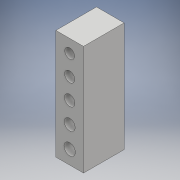
# Autodesk Inventor part: Screw size Test
Saved by Autodesk Inventor 2017 (Build 210142000, 142)
## iProperties
Created: 2017-05-18
Part Number: Screw size Test
Material: Generic
Document SubType Name: Modeling
Designer: Lillian
Density: 1 g/cm^3
Appearance: Default
Author: Lillian
Autodesk Inventor part; units mm, degrees
ref_plane "YZ Plane" through (0, 0, 0) normal (1, 0, 0) x (0, 1, 0)
ref_plane "XZ Plane" through (0, 0, 0) normal (0, 1, 0) x (-1, 0, 0)
ref_plane "XY Plane" through (0, 0, 0) normal (0, 0, 1) x (1, 0, 0)
sketch "Sketch1" plane through (0, 0, 0) normal (0, 1, 0) x (-1, 0, 0)
  circle A0 centre (0, 0) radius 1.3
  circle A1 centre (0, 5.05) radius 1.25
  circle A2 centre (0, -5.15) radius 1.35
  line L0 (3.4, 13.2) -> (-3.4, 13.2)
  line L1 (-3.4, 13.2) -> (-3.4, -13.8)
  line L2 (-3.4, -13.8) -> (3.4, -13.8)
  line L3 (3.4, -13.8) -> (3.4, 13.2)
  circle A3 centre (0, -10.4) radius 1.4
  circle A4 centre (0, 10) radius 1.2
  dimension "d0" = 2.6
  dimension "d1" = 2.5
  dimension "d2" = 2.5
  dimension "d3" = 2.5
  dimension "d4" = 2.7
  dimension "d5" = 2.5
  dimension "d6" = 2.5
  dimension "d7" = 2.8
  dimension "d8" = 2.4
  dimension "d9" = 2
  dimension "d10" = 2
  dimension "d11" = 2
  dimension "d12" = 2
  constraints: 8 end point, 5 centre point, 2 parallel, 1 coincident, 1 horizontal, 1 perpendicular
  measures "d0" diameter of A0
  measures "d3" diameter of A1
  measures "d4" diameter of A2
  measures "d7" diameter of A3
  measures "d8" diameter of A4
  measures "d9" distance edge to line of A3 L3
  measures "d10" distance edge to line of A3 L1
  measures "d11" distance edge to line of A3 L2
  measures "d12" distance edge to line of A4 L0
extrude "Extrusion1" add sketch "Sketch1" along normal blind 10
sketch "Sketch2" plane through (0, 10, 0) normal (0, 1, 0) x (1, 0, 0)
  line L0 (-2.0805, -11.7201) -> (2.1464, -11.7201) construction
  line L1 (2.1464, -11.7201) -> (2.1464, -12.7412) construction
  line L2 (2.1464, -12.7412) -> (-2.0805, -12.7412) construction
  line L3 (-2.0805, -12.7412) -> (-2.0805, -11.7201) construction
  line L4 (-1.0805, -10.7201) -> (3.1464, -10.7201) construction
  line L5 (3.1464, -10.7201) -> (3.1464, -11.7412) construction
  line L6 (3.1464, -11.7412) -> (-1.0805, -11.7412) construction
  line L7 (-1.0805, -11.7412) -> (-1.0805, -10.7201) construction
  line L8 (-1.8538, -6.831) -> (2.3732, -6.831) construction
  line L9 (2.3732, -6.831) -> (2.3732, -7.852) construction
  line L10 (2.3732, -7.852) -> (-1.8538, -7.852) construction
  line L11 (-1.8538, -7.852) -> (-1.8538, -6.831) construction
  line L12 (-1.9, -1.8736) -> (2.3269, -1.8736) construction
  line L13 (2.3269, -1.8736) -> (2.3269, -2.8947) construction
  line L14 (2.3269, -2.8947) -> (-1.9, -2.8947) construction
  line L15 (-1.9, -2.8947) -> (-1.9, -1.8736) construction
  line L16 (-1.934, 2.8467) -> (2.2929, 2.8467) construction
  line L17 (2.2929, 2.8467) -> (2.2929, 1.8257) construction
  line L18 (2.2929, 1.8257) -> (-1.934, 1.8257) construction
  line L19 (-1.934, 1.8257) -> (-1.934, 2.8467) construction
  line L20 (-1.7841, 8.3554) -> (2.4428, 8.3554) construction
  line L21 (2.4428, 8.3554) -> (2.4428, 7.3343) construction
  line L22 (2.4428, 7.3343) -> (-1.7841, 7.3343) construction
  line L23 (-1.7841, 7.3343) -> (-1.7841, 8.3554) construction
  line L24 (-1.3908, -12.7412) -> (-2.0075, -12.7412)
  line L25 (-2.0075, -12.7412) -> (-2.0075, -12.5994)
  spline S0 degree 2 poles (-2.0075, -12.5994) (-1.9411, -12.537) (-1.8228, -12.4211) (-1.766, -12.3587) knots 0 0 0 1 2 2 2
  spline S1 degree 2 poles (-1.766, -12.3587) (-1.6518, -12.2331) (-1.5683, -12.0824) (-1.5683, -12.0021) knots 0 0 0 1 2 2 2
  spline S2 degree 2 poles (-1.5683, -12.0021) (-1.5683, -11.96) (-1.5942, -11.8968) (-1.6177, -11.8765) knots 0 0 0 1 2 2 2
  spline S3 degree 2 poles (-1.6177, -11.8765) (-1.6413, -11.8563) (-1.7028, -11.836) (-1.7401, -11.836) knots 0 0 0 1 2 2 2
  spline S4 degree 2 poles (-1.7401, -11.836) (-1.7758, -11.836) (-1.8487, -11.8538) (-1.8819, -11.8676) knots 0 0 0 1 2 2 2
  spline S5 degree 2 poles (-1.8819, -11.8676) (-1.9103, -11.879) (-1.963, -11.9114) (-1.9792, -11.9227) knots 0 0 0 1 2 2 2
  line L26 (-1.9792, -11.9227) -> (-1.9865, -11.9227)
  line L27 (-1.9865, -11.9227) -> (-1.9865, -11.7801)
  spline S6 degree 2 poles (-1.9865, -11.7801) (-1.9451, -11.7598) (-1.7968, -11.7201) (-1.7304, -11.7201) knots 0 0 0 1 2 2 2
  spline S7 degree 2 poles (-1.7304, -11.7201) (-1.5902, -11.7201) (-1.4322, -11.8684) (-1.4322, -11.9948) knots 0 0 0 1 2 2 2
  spline S8 degree 2 poles (-1.4322, -11.9948) (-1.4322, -12.054) (-1.4597, -12.1529) (-1.484, -12.195) knots 0 0 0 1 2 2 2
  spline S9 degree 2 poles (-1.484, -12.195) (-1.5083, -12.2388) (-1.5789, -12.3247) (-1.6177, -12.366) knots 0 0 0 1 2 2 2
  spline S10 degree 2 poles (-1.6177, -12.366) (-1.681, -12.4349) (-1.8357, -12.5824) (-1.8819, -12.6253) knots 0 0 0 1 2 2 2
  line L28 (-1.8819, -12.6253) -> (-1.3908, -12.6253)
  line L29 (-1.3908, -12.6253) -> (-1.3908, -12.7412)
  line L30 (-1.0424, -12.7412) -> (-1.2028, -12.7412)
  line L31 (-1.2028, -12.7412) -> (-1.2028, -12.5499)
  line L32 (-1.2028, -12.5499) -> (-1.0424, -12.5499)
  line L33 (-1.0424, -12.5499) -> (-1.0424, -12.7412)
  line L34 (-0.1972, -12.3976) -> (-0.3163, -12.3976)
  line L35 (-0.3163, -12.3976) -> (-0.3163, -12.7412)
  line L36 (-0.3163, -12.7412) -> (-0.4451, -12.7412)
  line L37 (-0.4451, -12.7412) -> (-0.4451, -12.3976)
  line L38 (-0.4451, -12.3976) -> (-0.8868, -12.3976)
  line L39 (-0.8868, -12.3976) -> (-0.8868, -12.2566)
  line L40 (-0.8868, -12.2566) -> (-0.4395, -11.7412)
  line L41 (-0.4395, -11.7412) -> (-0.3163, -11.7412)
  line L42 (-0.3163, -11.7412) -> (-0.3163, -12.2898)
  line L43 (-0.3163, -12.2898) -> (-0.1972, -12.2898)
  line L44 (-0.1972, -12.2898) -> (-0.1972, -12.3976)
  line L45 (-0.4451, -12.2898) -> (-0.4451, -11.8992)
  line L46 (-0.4451, -11.8992) -> (-0.7814, -12.2898)
  line L47 (-0.7814, -12.2898) -> (-0.4451, -12.2898)
  line L48 (0.7793, -12.7412) -> (0.7793, -12.3068)
  spline S11 degree 2 poles (0.7793, -12.3068) (0.7793, -12.255) (0.7712, -12.1666) (0.7583, -12.1423) knots 0 0 0 1 2 2 2
  spline S12 degree 2 poles (0.7583, -12.1423) (0.7453, -12.1156) (0.6959, -12.0897) (0.6529, -12.0897) knots 0 0 0 1 2 2 2
  spline S13 degree 2 poles (0.6529, -12.0897) (0.614, -12.0897) (0.5249, -12.1375) (0.4779, -12.1828) knots 0 0 0 1 2 2 2
  spline S14 degree 2 poles (0.4779, -12.1828) (0.4787, -12.1942) (0.4803, -12.2258) (0.4803, -12.2469) knots 0 0 0 1 2 2 2
  line L49 (0.4803, -12.2469) -> (0.4803, -12.7412)
  line L50 (0.4803, -12.7412) -> (0.3539, -12.7412)
  line L51 (0.3539, -12.7412) -> (0.3539, -12.3068)
  spline S15 degree 2 poles (0.3539, -12.3068) (0.3539, -12.255) (0.3458, -12.1666) (0.3328, -12.1423) knots 0 0 0 1 2 2 2
  spline S16 degree 2 poles (0.3328, -12.1423) (0.3199, -12.1156) (0.2704, -12.0897) (0.2275, -12.0897) knots 0 0 0 1 2 2 2
  spline S17 degree 2 poles (0.2275, -12.0897) (0.187, -12.0897) (0.097, -12.1407) (0.0549, -12.1804) knots 0 0 0 1 2 2 2
  line L52 (0.0549, -12.1804) -> (0.0549, -12.7412)
  line L53 (0.0549, -12.7412) -> (-0.0716, -12.7412)
  line L54 (-0.0716, -12.7412) -> (-0.0716, -11.9908)
  line L55 (-0.0716, -11.9908) -> (0.0549, -11.9908)
  line L56 (0.0549, -11.9908) -> (0.0549, -12.0734)
  spline S18 degree 2 poles (0.0549, -12.0734) (0.1043, -12.024) (0.2015, -11.9697) (0.2599, -11.9697) knots 0 0 0 1 2 2 2
  spline S19 degree 2 poles (0.2599, -11.9697) (0.3263, -11.9697) (0.4293, -12.0305) (0.456, -12.0994) knots 0 0 0 1 2 2 2
  spline S20 degree 2 poles (0.456, -12.0994) (0.5135, -12.0354) (0.6221, -11.9697) (0.6853, -11.9697) knots 0 0 0 1 2 2 2
  spline S21 degree 2 poles (0.6853, -11.9697) (0.734, -11.9697) (0.8134, -11.9997) (0.8425, -12.0337) knots 0 0 0 1 2 2 2
  spline S22 degree 2 poles (0.8425, -12.0337) (0.8725, -12.0678) (0.9058, -12.1699) (0.9058, -12.2469) knots 0 0 0 1 2 2 2
  line L57 (0.9058, -12.2469) -> (0.9058, -12.7412)
  line L58 (0.9058, -12.7412) -> (0.7793, -12.7412)
  line L59 (1.9341, -12.7412) -> (1.9341, -12.3068)
  spline S23 degree 2 poles (1.9341, -12.3068) (1.9341, -12.255) (1.926, -12.1666) (1.913, -12.1423) knots 0 0 0 1 2 2 2
  spline S24 degree 2 poles (1.913, -12.1423) (1.9001, -12.1156) (1.8506, -12.0897) (1.8077, -12.0897) knots 0 0 0 1 2 2 2
  spline S25 degree 2 poles (1.8077, -12.0897) (1.7688, -12.0897) (1.6797, -12.1375) (1.6327, -12.1828) knots 0 0 0 1 2 2 2
  spline S26 degree 2 poles (1.6327, -12.1828) (1.6335, -12.1942) (1.6351, -12.2258) (1.6351, -12.2469) knots 0 0 0 1 2 2 2
  line L60 (1.6351, -12.2469) -> (1.6351, -12.7412)
  line L61 (1.6351, -12.7412) -> (1.5087, -12.7412)
  line L62 (1.5087, -12.7412) -> (1.5087, -12.3068)
  spline S27 degree 2 poles (1.5087, -12.3068) (1.5087, -12.255) (1.5006, -12.1666) (1.4876, -12.1423) knots 0 0 0 1 2 2 2
  spline S28 degree 2 poles (1.4876, -12.1423) (1.4746, -12.1156) (1.4252, -12.0897) (1.3823, -12.0897) knots 0 0 0 1 2 2 2
  spline S29 degree 2 poles (1.3823, -12.0897) (1.3417, -12.0897) (1.2518, -12.1407) (1.2096, -12.1804) knots 0 0 0 1 2 2 2
  line L63 (1.2096, -12.1804) -> (1.2096, -12.7412)
  line L64 (1.2096, -12.7412) -> (1.0832, -12.7412)
  line L65 (1.0832, -12.7412) -> (1.0832, -11.9908)
  line L66 (1.0832, -11.9908) -> (1.2096, -11.9908)
  line L67 (1.2096, -11.9908) -> (1.2096, -12.0734)
  spline S30 degree 2 poles (1.2096, -12.0734) (1.2591, -12.024) (1.3563, -11.9697) (1.4147, -11.9697) knots 0 0 0 1 2 2 2
  spline S31 degree 2 poles (1.4147, -11.9697) (1.4811, -11.9697) (1.584, -12.0305) (1.6108, -12.0994) knots 0 0 0 1 2 2 2
  spline S32 degree 2 poles (1.6108, -12.0994) (1.6683, -12.0354) (1.7769, -11.9697) (1.8401, -11.9697) knots 0 0 0 1 2 2 2
  spline S33 degree 2 poles (1.8401, -11.9697) (1.8887, -11.9697) (1.9682, -11.9997) (1.9973, -12.0337) knots 0 0 0 1 2 2 2
  spline S34 degree 2 poles (1.9973, -12.0337) (2.0273, -12.0678) (2.0605, -12.1699) (2.0605, -12.2469) knots 0 0 0 1 2 2 2
  line L68 (2.0605, -12.2469) -> (2.0605, -12.7412)
  line L69 (2.0605, -12.7412) -> (1.9341, -12.7412)
  line L70 (-1.1641, -7.852) -> (-1.7808, -7.852)
  line L71 (-1.7808, -7.852) -> (-1.7808, -7.7102)
  spline S35 degree 2 poles (-1.7808, -7.7102) (-1.7144, -7.6478) (-1.5961, -7.5319) (-1.5393, -7.4695) knots 0 0 0 1 2 2 2
  spline S36 degree 2 poles (-1.5393, -7.4695) (-1.4251, -7.3439) (-1.3416, -7.1932) (-1.3416, -7.113) knots 0 0 0 1 2 2 2
  spline S37 degree 2 poles (-1.3416, -7.113) (-1.3416, -7.0708) (-1.3675, -7.0076) (-1.391, -6.9874) knots 0 0 0 1 2 2 2
  spline S38 degree 2 poles (-1.391, -6.9874) (-1.4145, -6.9671) (-1.4761, -6.9469) (-1.5134, -6.9469) knots 0 0 0 1 2 2 2
  spline S39 degree 2 poles (-1.5134, -6.9469) (-1.5491, -6.9469) (-1.622, -6.9647) (-1.6552, -6.9785) knots 0 0 0 1 2 2 2
  spline S40 degree 2 poles (-1.6552, -6.9785) (-1.6836, -6.9898) (-1.7363, -7.0222) (-1.7525, -7.0336) knots 0 0 0 1 2 2 2
  line L72 (-1.7525, -7.0336) -> (-1.7598, -7.0336)
  line L73 (-1.7598, -7.0336) -> (-1.7598, -6.8909)
  spline S41 degree 2 poles (-1.7598, -6.8909) (-1.7184, -6.8707) (-1.5701, -6.831) (-1.5037, -6.831) knots 0 0 0 1 2 2 2
  spline S42 degree 2 poles (-1.5037, -6.831) (-1.3635, -6.831) (-1.2055, -6.9793) (-1.2055, -7.1057) knots 0 0 0 1 2 2 2
  spline S43 degree 2 poles (-1.2055, -7.1057) (-1.2055, -7.1648) (-1.233, -7.2637) (-1.2573, -7.3058) knots 0 0 0 1 2 2 2
  spline S44 degree 2 poles (-1.2573, -7.3058) (-1.2816, -7.3496) (-1.3521, -7.4355) (-1.391, -7.4768) knots 0 0 0 1 2 2 2
  spline S45 degree 2 poles (-1.391, -7.4768) (-1.4542, -7.5457) (-1.609, -7.6932) (-1.6552, -7.7362) knots 0 0 0 1 2 2 2
  line L74 (-1.6552, -7.7362) -> (-1.1641, -7.7362)
  line L75 (-1.1641, -7.7362) -> (-1.1641, -7.852)
  line L76 (-0.8157, -7.852) -> (-0.9761, -7.852)
  line L77 (-0.9761, -7.852) -> (-0.9761, -7.6608)
  line L78 (-0.9761, -7.6608) -> (-0.8157, -7.6608)
  line L79 (-0.8157, -7.6608) -> (-0.8157, -7.852)
  spline S46 degree 2 poles (-0.0077, -7.5344) (-0.0077, -7.6065) (-0.0539, -7.7297) (-0.0961, -7.7751) knots 0 0 0 1 2 2 2
  spline S47 degree 2 poles (-0.0961, -7.7751) (-0.1382, -7.8204) (-0.2638, -7.8731) (-0.3416, -7.8731) knots 0 0 0 1 2 2 2
  spline S48 degree 2 poles (-0.3416, -7.8731) (-0.4129, -7.8731) (-0.5523, -7.8415) (-0.6033, -7.8164) knots 0 0 0 1 2 2 2
  line L80 (-0.6033, -7.8164) -> (-0.6033, -7.6746)
  line L81 (-0.6033, -7.6746) -> (-0.5936, -7.6746)
  spline S49 degree 2 poles (-0.5936, -7.6746) (-0.5782, -7.6859) (-0.5207, -7.7151) (-0.4858, -7.7281) knots 0 0 0 1 2 2 2
  spline S50 degree 2 poles (-0.4858, -7.7281) (-0.4461, -7.7418) (-0.3805, -7.7572) (-0.3392, -7.7572) knots 0 0 0 1 2 2 2
  spline S51 degree 2 poles (-0.3392, -7.7572) (-0.2986, -7.7572) (-0.2225, -7.7281) (-0.1949, -7.6964) knots 0 0 0 1 2 2 2
  spline S52 degree 2 poles (-0.1949, -7.6964) (-0.1698, -7.6665) (-0.1439, -7.587) (-0.1439, -7.5336) knots 0 0 0 1 2 2 2
  spline S53 degree 2 poles (-0.1439, -7.5336) (-0.1439, -7.4801) (-0.173, -7.412) (-0.2006, -7.3893) knots 0 0 0 1 2 2 2
  spline S54 degree 2 poles (-0.2006, -7.3893) (-0.229, -7.3642) (-0.3132, -7.3431) (-0.3643, -7.3431) knots 0 0 0 1 2 2 2
  spline S55 degree 2 poles (-0.3643, -7.3431) (-0.4194, -7.3431) (-0.5288, -7.3601) (-0.562, -7.3674) knots 0 0 0 1 2 2 2
  line L82 (-0.562, -7.3674) -> (-0.562, -6.852)
  line L83 (-0.562, -6.852) -> (-0.0134, -6.852)
  line L84 (-0.0134, -6.852) -> (-0.0134, -6.9695)
  line L85 (-0.0134, -6.9695) -> (-0.4332, -6.9695)
  line L86 (-0.4332, -6.9695) -> (-0.4332, -7.2362)
  spline S56 degree 2 poles (-0.4332, -7.2362) (-0.4089, -7.2329) (-0.3619, -7.2305) (-0.3424, -7.2305) knots 0 0 0 1 2 2 2
  spline S57 degree 2 poles (-0.3424, -7.2305) (-0.2654, -7.2305) (-0.1593, -7.2556) (-0.1106, -7.2929) knots 0 0 0 1 2 2 2
  spline S58 degree 2 poles (-0.1106, -7.2929) (-0.0612, -7.3302) (-0.0077, -7.4436) (-0.0077, -7.5344) knots 0 0 0 1 2 2 2
  line L87 (1.0061, -7.852) -> (1.0061, -7.4177)
  spline S59 degree 2 poles (1.0061, -7.4177) (1.0061, -7.3658) (0.9979, -7.2775) (0.985, -7.2532) knots 0 0 0 1 2 2 2
  spline S60 degree 2 poles (0.985, -7.2532) (0.972, -7.2264) (0.9226, -7.2005) (0.8796, -7.2005) knots 0 0 0 1 2 2 2
  spline S61 degree 2 poles (0.8796, -7.2005) (0.8407, -7.2005) (0.7516, -7.2483) (0.7046, -7.2937) knots 0 0 0 1 2 2 2
  spline S62 degree 2 poles (0.7046, -7.2937) (0.7054, -7.305) (0.707, -7.3366) (0.707, -7.3577) knots 0 0 0 1 2 2 2
  line L88 (0.707, -7.3577) -> (0.707, -7.852)
  line L89 (0.707, -7.852) -> (0.5806, -7.852)
  line L90 (0.5806, -7.852) -> (0.5806, -7.4177)
  spline S63 degree 2 poles (0.5806, -7.4177) (0.5806, -7.3658) (0.5725, -7.2775) (0.5595, -7.2532) knots 0 0 0 1 2 2 2
  spline S64 degree 2 poles (0.5595, -7.2532) (0.5466, -7.2264) (0.4971, -7.2005) (0.4542, -7.2005) knots 0 0 0 1 2 2 2
  spline S65 degree 2 poles (0.4542, -7.2005) (0.4137, -7.2005) (0.3237, -7.2516) (0.2816, -7.2913) knots 0 0 0 1 2 2 2
  line L91 (0.2816, -7.2913) -> (0.2816, -7.852)
  line L92 (0.2816, -7.852) -> (0.1552, -7.852)
  line L93 (0.1552, -7.852) -> (0.1552, -7.1016)
  line L94 (0.1552, -7.1016) -> (0.2816, -7.1016)
  line L95 (0.2816, -7.1016) -> (0.2816, -7.1843)
  spline S66 degree 2 poles (0.2816, -7.1843) (0.331, -7.1349) (0.4283, -7.0806) (0.4866, -7.0806) knots 0 0 0 1 2 2 2
  spline S67 degree 2 poles (0.4866, -7.0806) (0.5531, -7.0806) (0.656, -7.1413) (0.6827, -7.2102) knots 0 0 0 1 2 2 2
  spline S68 degree 2 poles (0.6827, -7.2102) (0.7402, -7.1462) (0.8488, -7.0806) (0.912, -7.0806) knots 0 0 0 1 2 2 2
  spline S69 degree 2 poles (0.912, -7.0806) (0.9607, -7.0806) (1.0401, -7.1105) (1.0693, -7.1446) knots 0 0 0 1 2 2 2
  spline S70 degree 2 poles (1.0693, -7.1446) (1.0992, -7.1786) (1.1325, -7.2807) (1.1325, -7.3577) knots 0 0 0 1 2 2 2
  line L96 (1.1325, -7.3577) -> (1.1325, -7.852)
  line L97 (1.1325, -7.852) -> (1.0061, -7.852)
  line L98 (2.1608, -7.852) -> (2.1608, -7.4177)
  spline S71 degree 2 poles (2.1608, -7.4177) (2.1608, -7.3658) (2.1527, -7.2775) (2.1398, -7.2532) knots 0 0 0 1 2 2 2
  spline S72 degree 2 poles (2.1398, -7.2532) (2.1268, -7.2264) (2.0774, -7.2005) (2.0344, -7.2005) knots 0 0 0 1 2 2 2
  spline S73 degree 2 poles (2.0344, -7.2005) (1.9955, -7.2005) (1.9064, -7.2483) (1.8594, -7.2937) knots 0 0 0 1 2 2 2
  spline S74 degree 2 poles (1.8594, -7.2937) (1.8602, -7.305) (1.8618, -7.3366) (1.8618, -7.3577) knots 0 0 0 1 2 2 2
  line L99 (1.8618, -7.3577) -> (1.8618, -7.852)
  line L100 (1.8618, -7.852) -> (1.7354, -7.852)
  line L101 (1.7354, -7.852) -> (1.7354, -7.4177)
  spline S75 degree 2 poles (1.7354, -7.4177) (1.7354, -7.3658) (1.7273, -7.2775) (1.7143, -7.2532) knots 0 0 0 1 2 2 2
  spline S76 degree 2 poles (1.7143, -7.2532) (1.7014, -7.2264) (1.6519, -7.2005) (1.609, -7.2005) knots 0 0 0 1 2 2 2
  spline S77 degree 2 poles (1.609, -7.2005) (1.5685, -7.2005) (1.4785, -7.2516) (1.4364, -7.2913) knots 0 0 0 1 2 2 2
  line L102 (1.4364, -7.2913) -> (1.4364, -7.852)
  line L103 (1.4364, -7.852) -> (1.3099, -7.852)
  line L104 (1.3099, -7.852) -> (1.3099, -7.1016)
  line L105 (1.3099, -7.1016) -> (1.4364, -7.1016)
  line L106 (1.4364, -7.1016) -> (1.4364, -7.1843)
  spline S78 degree 2 poles (1.4364, -7.1843) (1.4858, -7.1349) (1.583, -7.0806) (1.6414, -7.0806) knots 0 0 0 1 2 2 2
  spline S79 degree 2 poles (1.6414, -7.0806) (1.7078, -7.0806) (1.8108, -7.1413) (1.8375, -7.2102) knots 0 0 0 1 2 2 2
  spline S80 degree 2 poles (1.8375, -7.2102) (1.895, -7.1462) (2.0036, -7.0806) (2.0668, -7.0806) knots 0 0 0 1 2 2 2
  spline S81 degree 2 poles (2.0668, -7.0806) (2.1155, -7.0806) (2.1949, -7.1105) (2.224, -7.1446) knots 0 0 0 1 2 2 2
  spline S82 degree 2 poles (2.224, -7.1446) (2.254, -7.1786) (2.2873, -7.2807) (2.2873, -7.3577) knots 0 0 0 1 2 2 2
  line L107 (2.2873, -7.3577) -> (2.2873, -7.852)
  line L108 (2.2873, -7.852) -> (2.1608, -7.852)
  line L109 (-1.2103, -2.8947) -> (-1.827, -2.8947)
  line L110 (-1.827, -2.8947) -> (-1.827, -2.7528)
  spline S83 degree 2 poles (-1.827, -2.7528) (-1.7606, -2.6904) (-1.6423, -2.5746) (-1.5855, -2.5122) knots 0 0 0 1 2 2 2
  spline S84 degree 2 poles (-1.5855, -2.5122) (-1.4713, -2.3866) (-1.3878, -2.2358) (-1.3878, -2.1556) knots 0 0 0 1 2 2 2
  spline S85 degree 2 poles (-1.3878, -2.1556) (-1.3878, -2.1135) (-1.4137, -2.0502) (-1.4372, -2.03) knots 0 0 0 1 2 2 2
  spline S86 degree 2 poles (-1.4372, -2.03) (-1.4607, -2.0097) (-1.5223, -1.9895) (-1.5596, -1.9895) knots 0 0 0 1 2 2 2
  spline S87 degree 2 poles (-1.5596, -1.9895) (-1.5953, -1.9895) (-1.6682, -2.0073) (-1.7014, -2.0211) knots 0 0 0 1 2 2 2
  spline S88 degree 2 poles (-1.7014, -2.0211) (-1.7298, -2.0324) (-1.7825, -2.0648) (-1.7987, -2.0762) knots 0 0 0 1 2 2 2
  line L111 (-1.7987, -2.0762) -> (-1.806, -2.0762)
  line L112 (-1.806, -2.0762) -> (-1.806, -1.9336)
  spline S89 degree 2 poles (-1.806, -1.9336) (-1.7646, -1.9133) (-1.6163, -1.8736) (-1.5499, -1.8736) knots 0 0 0 1 2 2 2
  spline S90 degree 2 poles (-1.5499, -1.8736) (-1.4097, -1.8736) (-1.2517, -2.0219) (-1.2517, -2.1483) knots 0 0 0 1 2 2 2
  spline S91 degree 2 poles (-1.2517, -2.1483) (-1.2517, -2.2075) (-1.2792, -2.3063) (-1.3035, -2.3485) knots 0 0 0 1 2 2 2
  spline S92 degree 2 poles (-1.3035, -2.3485) (-1.3278, -2.3922) (-1.3983, -2.4781) (-1.4372, -2.5195) knots 0 0 0 1 2 2 2
  spline S93 degree 2 poles (-1.4372, -2.5195) (-1.5004, -2.5883) (-1.6552, -2.7358) (-1.7014, -2.7788) knots 0 0 0 1 2 2 2
  line L113 (-1.7014, -2.7788) -> (-1.2103, -2.7788)
  line L114 (-1.2103, -2.7788) -> (-1.2103, -2.8947)
  line L115 (-0.8619, -2.8947) -> (-1.0223, -2.8947)
  line L116 (-1.0223, -2.8947) -> (-1.0223, -2.7034)
  line L117 (-1.0223, -2.7034) -> (-0.8619, -2.7034)
  line L118 (-0.8619, -2.7034) -> (-0.8619, -2.8947)
  spline S94 degree 2 poles (-0.028, -2.5705) (-0.028, -2.6475) (-0.0791, -2.778) (-0.122, -2.8217) knots 0 0 0 1 2 2 2
  spline S95 degree 2 poles (-0.122, -2.8217) (-0.1666, -2.8679) (-0.2784, -2.9157) (-0.3457, -2.9157) knots 0 0 0 1 2 2 2
  spline S96 degree 2 poles (-0.3457, -2.9157) (-0.4129, -2.9157) (-0.5239, -2.8703) (-0.5661, -2.825) knots 0 0 0 1 2 2 2
  spline S97 degree 2 poles (-0.5661, -2.825) (-0.6179, -2.7707) (-0.6763, -2.5883) (-0.6763, -2.4554) knots 0 0 0 1 2 2 2
  spline S98 degree 2 poles (-0.6763, -2.4554) (-0.6763, -2.325) (-0.6228, -2.1151) (-0.5669, -2.0373) knots 0 0 0 1 2 2 2
  spline S99 degree 2 poles (-0.5669, -2.0373) (-0.5126, -1.9611) (-0.3408, -1.876) (-0.2282, -1.876) knots 0 0 0 1 2 2 2
  spline S100 degree 2 poles (-0.2282, -1.876) (-0.1949, -1.876) (-0.1366, -1.8825) (-0.1147, -1.8898) knots 0 0 0 1 2 2 2
  line L119 (-0.1147, -1.8898) -> (-0.1147, -2.0186)
  line L120 (-0.1147, -2.0186) -> (-0.1204, -2.0186)
  spline S101 degree 2 poles (-0.1204, -2.0186) (-0.139, -2.0089) (-0.2071, -1.9919) (-0.246, -1.9919) knots 0 0 0 1 2 2 2
  spline S102 degree 2 poles (-0.246, -1.9919) (-0.3708, -1.9919) (-0.5239, -2.1605) (-0.5385, -2.3258) knots 0 0 0 1 2 2 2
  spline S103 degree 2 poles (-0.5385, -2.3258) (-0.4907, -2.2925) (-0.3902, -2.2561) (-0.3303, -2.2561) knots 0 0 0 1 2 2 2
  spline S104 degree 2 poles (-0.3303, -2.2561) (-0.2719, -2.2561) (-0.1844, -2.2796) (-0.1366, -2.3152) knots 0 0 0 1 2 2 2
  spline S105 degree 2 poles (-0.1366, -2.3152) (-0.0815, -2.3566) (-0.028, -2.4846) (-0.028, -2.5705) knots 0 0 0 1 2 2 2
  spline S106 degree 2 poles (-0.1641, -2.5762) (-0.1641, -2.5146) (-0.1966, -2.4311) (-0.2322, -2.4019) knots 0 0 0 1 2 2 2
  spline S107 degree 2 poles (-0.2322, -2.4019) (-0.259, -2.3809) (-0.3254, -2.3671) (-0.3603, -2.3671) knots 0 0 0 1 2 2 2
  spline S108 degree 2 poles (-0.3603, -2.3671) (-0.4073, -2.3671) (-0.4956, -2.3955) (-0.5385, -2.4222) knots 0 0 0 1 2 2 2
  spline S109 degree 2 poles (-0.5385, -2.4222) (-0.5393, -2.4368) (-0.541, -2.4643) (-0.541, -2.4854) knots 0 0 0 1 2 2 2
  spline S110 degree 2 poles (-0.541, -2.4854) (-0.541, -2.5891) (-0.5004, -2.7164) (-0.4697, -2.7496) knots 0 0 0 1 2 2 2
  spline S111 degree 2 poles (-0.4697, -2.7496) (-0.4413, -2.7812) (-0.3797, -2.8063) (-0.3449, -2.8063) knots 0 0 0 1 2 2 2
  spline S112 degree 2 poles (-0.3449, -2.8063) (-0.2638, -2.8063) (-0.1641, -2.6913) (-0.1641, -2.5762) knots 0 0 0 1 2 2 2
  line L121 (0.9598, -2.8947) -> (0.9598, -2.4603)
  spline S113 degree 2 poles (0.9598, -2.4603) (0.9598, -2.4084) (0.9517, -2.3201) (0.9388, -2.2958) knots 0 0 0 1 2 2 2
  spline S114 degree 2 poles (0.9388, -2.2958) (0.9258, -2.269) (0.8764, -2.2431) (0.8334, -2.2431) knots 0 0 0 1 2 2 2
  spline S115 degree 2 poles (0.8334, -2.2431) (0.7945, -2.2431) (0.7054, -2.2909) (0.6584, -2.3363) knots 0 0 0 1 2 2 2
  spline S116 degree 2 poles (0.6584, -2.3363) (0.6592, -2.3477) (0.6608, -2.3793) (0.6608, -2.4003) knots 0 0 0 1 2 2 2
  line L122 (0.6608, -2.4003) -> (0.6608, -2.8947)
  line L123 (0.6608, -2.8947) -> (0.5344, -2.8947)
  line L124 (0.5344, -2.8947) -> (0.5344, -2.4603)
  spline S117 degree 2 poles (0.5344, -2.4603) (0.5344, -2.4084) (0.5263, -2.3201) (0.5133, -2.2958) knots 0 0 0 1 2 2 2
  spline S118 degree 2 poles (0.5133, -2.2958) (0.5004, -2.269) (0.4509, -2.2431) (0.408, -2.2431) knots 0 0 0 1 2 2 2
  spline S119 degree 2 poles (0.408, -2.2431) (0.3675, -2.2431) (0.2775, -2.2942) (0.2354, -2.3339) knots 0 0 0 1 2 2 2
  line L125 (0.2354, -2.3339) -> (0.2354, -2.8947)
  line L126 (0.2354, -2.8947) -> (0.109, -2.8947)
  line L127 (0.109, -2.8947) -> (0.109, -2.1443)
  line L128 (0.109, -2.1443) -> (0.2354, -2.1443)
  line L129 (0.2354, -2.1443) -> (0.2354, -2.2269)
  spline S120 degree 2 poles (0.2354, -2.2269) (0.2848, -2.1775) (0.3821, -2.1232) (0.4404, -2.1232) knots 0 0 0 1 2 2 2
  spline S121 degree 2 poles (0.4404, -2.1232) (0.5068, -2.1232) (0.6098, -2.184) (0.6365, -2.2528) knots 0 0 0 1 2 2 2
  spline S122 degree 2 poles (0.6365, -2.2528) (0.694, -2.1888) (0.8026, -2.1232) (0.8658, -2.1232) knots 0 0 0 1 2 2 2
  spline S123 degree 2 poles (0.8658, -2.1232) (0.9145, -2.1232) (0.9939, -2.1532) (1.0231, -2.1872) knots 0 0 0 1 2 2 2
  spline S124 degree 2 poles (1.0231, -2.1872) (1.053, -2.2212) (1.0863, -2.3233) (1.0863, -2.4003) knots 0 0 0 1 2 2 2
  line L130 (1.0863, -2.4003) -> (1.0863, -2.8947)
  line L131 (1.0863, -2.8947) -> (0.9598, -2.8947)
  line L132 (2.1146, -2.8947) -> (2.1146, -2.4603)
  spline S125 degree 2 poles (2.1146, -2.4603) (2.1146, -2.4084) (2.1065, -2.3201) (2.0936, -2.2958) knots 0 0 0 1 2 2 2
  spline S126 degree 2 poles (2.0936, -2.2958) (2.0806, -2.269) (2.0312, -2.2431) (1.9882, -2.2431) knots 0 0 0 1 2 2 2
  spline S127 degree 2 poles (1.9882, -2.2431) (1.9493, -2.2431) (1.8602, -2.2909) (1.8132, -2.3363) knots 0 0 0 1 2 2 2
  spline S128 degree 2 poles (1.8132, -2.3363) (1.814, -2.3477) (1.8156, -2.3793) (1.8156, -2.4003) knots 0 0 0 1 2 2 2
  line L133 (1.8156, -2.4003) -> (1.8156, -2.8947)
  line L134 (1.8156, -2.8947) -> (1.6892, -2.8947)
  line L135 (1.6892, -2.8947) -> (1.6892, -2.4603)
  spline S129 degree 2 poles (1.6892, -2.4603) (1.6892, -2.4084) (1.6811, -2.3201) (1.6681, -2.2958) knots 0 0 0 1 2 2 2
  spline S130 degree 2 poles (1.6681, -2.2958) (1.6551, -2.269) (1.6057, -2.2431) (1.5628, -2.2431) knots 0 0 0 1 2 2 2
  spline S131 degree 2 poles (1.5628, -2.2431) (1.5222, -2.2431) (1.4323, -2.2942) (1.3902, -2.3339) knots 0 0 0 1 2 2 2
  line L136 (1.3902, -2.3339) -> (1.3902, -2.8947)
  line L137 (1.3902, -2.8947) -> (1.2637, -2.8947)
  line L138 (1.2637, -2.8947) -> (1.2637, -2.1443)
  line L139 (1.2637, -2.1443) -> (1.3902, -2.1443)
  line L140 (1.3902, -2.1443) -> (1.3902, -2.2269)
  spline S132 degree 2 poles (1.3902, -2.2269) (1.4396, -2.1775) (1.5368, -2.1232) (1.5952, -2.1232) knots 0 0 0 1 2 2 2
  spline S133 degree 2 poles (1.5952, -2.1232) (1.6616, -2.1232) (1.7645, -2.184) (1.7913, -2.2528) knots 0 0 0 1 2 2 2
  spline S134 degree 2 poles (1.7913, -2.2528) (1.8488, -2.1888) (1.9574, -2.1232) (2.0206, -2.1232) knots 0 0 0 1 2 2 2
  spline S135 degree 2 poles (2.0206, -2.1232) (2.0692, -2.1232) (2.1487, -2.1532) (2.1778, -2.1872) knots 0 0 0 1 2 2 2
  spline S136 degree 2 poles (2.1778, -2.1872) (2.2078, -2.2212) (2.241, -2.3233) (2.241, -2.4003) knots 0 0 0 1 2 2 2
  line L141 (2.241, -2.4003) -> (2.241, -2.8947)
  line L142 (2.241, -2.8947) -> (2.1146, -2.8947)
  line L143 (-1.2444, 1.8257) -> (-1.8611, 1.8257)
  line L144 (-1.8611, 1.8257) -> (-1.8611, 1.9675)
  spline S137 degree 2 poles (-1.8611, 1.9675) (-1.7946, 2.0299) (-1.6763, 2.1458) (-1.6196, 2.2082) knots 0 0 0 1 2 2 2
  spline S138 degree 2 poles (-1.6196, 2.2082) (-1.5053, 2.3338) (-1.4218, 2.4845) (-1.4218, 2.5647) knots 0 0 0 1 2 2 2
  spline S139 degree 2 poles (-1.4218, 2.5647) (-1.4218, 2.6069) (-1.4478, 2.6701) (-1.4713, 2.6903) knots 0 0 0 1 2 2 2
  spline S140 degree 2 poles (-1.4713, 2.6903) (-1.4948, 2.7106) (-1.5564, 2.7309) (-1.5936, 2.7309) knots 0 0 0 1 2 2 2
  spline S141 degree 2 poles (-1.5936, 2.7309) (-1.6293, 2.7309) (-1.7022, 2.713) (-1.7354, 2.6993) knots 0 0 0 1 2 2 2
  spline S142 degree 2 poles (-1.7354, 2.6993) (-1.7638, 2.6879) (-1.8165, 2.6555) (-1.8327, 2.6442) knots 0 0 0 1 2 2 2
  line L145 (-1.8327, 2.6442) -> (-1.84, 2.6442)
  line L146 (-1.84, 2.6442) -> (-1.84, 2.7868)
  spline S143 degree 2 poles (-1.84, 2.7868) (-1.7987, 2.807) (-1.6504, 2.8467) (-1.5839, 2.8467) knots 0 0 0 1 2 2 2
  spline S144 degree 2 poles (-1.5839, 2.8467) (-1.4437, 2.8467) (-1.2857, 2.6984) (-1.2857, 2.572) knots 0 0 0 1 2 2 2
  spline S145 degree 2 poles (-1.2857, 2.572) (-1.2857, 2.5129) (-1.3132, 2.414) (-1.3376, 2.3719) knots 0 0 0 1 2 2 2
  spline S146 degree 2 poles (-1.3376, 2.3719) (-1.3619, 2.3281) (-1.4324, 2.2422) (-1.4713, 2.2009) knots 0 0 0 1 2 2 2
  spline S147 degree 2 poles (-1.4713, 2.2009) (-1.5345, 2.132) (-1.6893, 1.9845) (-1.7354, 1.9416) knots 0 0 0 1 2 2 2
  line L147 (-1.7354, 1.9416) -> (-1.2444, 1.9416)
  line L148 (-1.2444, 1.9416) -> (-1.2444, 1.8257)
  line L149 (-0.8959, 1.8257) -> (-1.0564, 1.8257)
  line L150 (-1.0564, 1.8257) -> (-1.0564, 2.0169)
  line L151 (-1.0564, 2.0169) -> (-0.8959, 2.0169)
  line L152 (-0.8959, 2.0169) -> (-0.8959, 1.8257)
  line L153 (-0.0661, 2.6758) -> (-0.4988, 1.8257)
  line L154 (-0.4988, 1.8257) -> (-0.6414, 1.8257)
  line L155 (-0.6414, 1.8257) -> (-0.1844, 2.7082)
  line L156 (-0.1844, 2.7082) -> (-0.7006, 2.7082)
  line L157 (-0.7006, 2.7082) -> (-0.7006, 2.8257)
  line L158 (-0.7006, 2.8257) -> (-0.0661, 2.8257)
  line L159 (-0.0661, 2.8257) -> (-0.0661, 2.6758)
  line L160 (0.9258, 1.8257) -> (0.9258, 2.26)
  spline S148 degree 2 poles (0.9258, 2.26) (0.9258, 2.3119) (0.9177, 2.4002) (0.9047, 2.4245) knots 0 0 0 1 2 2 2
  spline S149 degree 2 poles (0.9047, 2.4245) (0.8918, 2.4513) (0.8423, 2.4772) (0.7994, 2.4772) knots 0 0 0 1 2 2 2
  spline S150 degree 2 poles (0.7994, 2.4772) (0.7605, 2.4772) (0.6714, 2.4294) (0.6244, 2.384) knots 0 0 0 1 2 2 2
  spline S151 degree 2 poles (0.6244, 2.384) (0.6252, 2.3727) (0.6268, 2.3411) (0.6268, 2.32) knots 0 0 0 1 2 2 2
  line L161 (0.6268, 2.32) -> (0.6268, 1.8257)
  line L162 (0.6268, 1.8257) -> (0.5004, 1.8257)
  line L163 (0.5004, 1.8257) -> (0.5004, 2.26)
  spline S152 degree 2 poles (0.5004, 2.26) (0.5004, 2.3119) (0.4923, 2.4002) (0.4793, 2.4245) knots 0 0 0 1 2 2 2
  spline S153 degree 2 poles (0.4793, 2.4245) (0.4663, 2.4513) (0.4169, 2.4772) (0.374, 2.4772) knots 0 0 0 1 2 2 2
  spline S154 degree 2 poles (0.374, 2.4772) (0.3334, 2.4772) (0.2435, 2.4262) (0.2013, 2.3865) knots 0 0 0 1 2 2 2
  line L164 (0.2013, 2.3865) -> (0.2013, 1.8257)
  line L165 (0.2013, 1.8257) -> (0.0749, 1.8257)
  line L166 (0.0749, 1.8257) -> (0.0749, 2.5761)
  line L167 (0.0749, 2.5761) -> (0.2013, 2.5761)
  line L168 (0.2013, 2.5761) -> (0.2013, 2.4934)
  spline S155 degree 2 poles (0.2013, 2.4934) (0.2508, 2.5429) (0.348, 2.5972) (0.4064, 2.5972) knots 0 0 0 1 2 2 2
  spline S156 degree 2 poles (0.4064, 2.5972) (0.4728, 2.5972) (0.5757, 2.5364) (0.6025, 2.4675) knots 0 0 0 1 2 2 2
  spline S157 degree 2 poles (0.6025, 2.4675) (0.66, 2.5315) (0.7686, 2.5972) (0.8318, 2.5972) knots 0 0 0 1 2 2 2
  spline S158 degree 2 poles (0.8318, 2.5972) (0.8804, 2.5972) (0.9599, 2.5672) (0.989, 2.5331) knots 0 0 0 1 2 2 2
  spline S159 degree 2 poles (0.989, 2.5331) (1.019, 2.4991) (1.0522, 2.397) (1.0522, 2.32) knots 0 0 0 1 2 2 2
  line L169 (1.0522, 2.32) -> (1.0522, 1.8257)
  line L170 (1.0522, 1.8257) -> (0.9258, 1.8257)
  line L171 (2.0806, 1.8257) -> (2.0806, 2.26)
  spline S160 degree 2 poles (2.0806, 2.26) (2.0806, 2.3119) (2.0725, 2.4002) (2.0595, 2.4245) knots 0 0 0 1 2 2 2
  spline S161 degree 2 poles (2.0595, 2.4245) (2.0466, 2.4513) (1.9971, 2.4772) (1.9542, 2.4772) knots 0 0 0 1 2 2 2
  spline S162 degree 2 poles (1.9542, 2.4772) (1.9153, 2.4772) (1.8261, 2.4294) (1.7791, 2.384) knots 0 0 0 1 2 2 2
  spline S163 degree 2 poles (1.7791, 2.384) (1.7799, 2.3727) (1.7816, 2.3411) (1.7816, 2.32) knots 0 0 0 1 2 2 2
  line L172 (1.7816, 2.32) -> (1.7816, 1.8257)
  line L173 (1.7816, 1.8257) -> (1.6552, 1.8257)
  line L174 (1.6552, 1.8257) -> (1.6552, 2.26)
  spline S164 degree 2 poles (1.6552, 2.26) (1.6552, 2.3119) (1.647, 2.4002) (1.6341, 2.4245) knots 0 0 0 1 2 2 2
  spline S165 degree 2 poles (1.6341, 2.4245) (1.6211, 2.4513) (1.5717, 2.4772) (1.5287, 2.4772) knots 0 0 0 1 2 2 2
  spline S166 degree 2 poles (1.5287, 2.4772) (1.4882, 2.4772) (1.3983, 2.4262) (1.3561, 2.3865) knots 0 0 0 1 2 2 2
  line L175 (1.3561, 2.3865) -> (1.3561, 1.8257)
  line L176 (1.3561, 1.8257) -> (1.2297, 1.8257)
  line L177 (1.2297, 1.8257) -> (1.2297, 2.5761)
  line L178 (1.2297, 2.5761) -> (1.3561, 2.5761)
  line L179 (1.3561, 2.5761) -> (1.3561, 2.4934)
  spline S167 degree 2 poles (1.3561, 2.4934) (1.4056, 2.5429) (1.5028, 2.5972) (1.5611, 2.5972) knots 0 0 0 1 2 2 2
  spline S168 degree 2 poles (1.5611, 2.5972) (1.6276, 2.5972) (1.7305, 2.5364) (1.7573, 2.4675) knots 0 0 0 1 2 2 2
  spline S169 degree 2 poles (1.7573, 2.4675) (1.8148, 2.5315) (1.9234, 2.5972) (1.9866, 2.5972) knots 0 0 0 1 2 2 2
  spline S170 degree 2 poles (1.9866, 2.5972) (2.0352, 2.5972) (2.1146, 2.5672) (2.1438, 2.5331) knots 0 0 0 1 2 2 2
  spline S171 degree 2 poles (2.1438, 2.5331) (2.1738, 2.4991) (2.207, 2.397) (2.207, 2.32) knots 0 0 0 1 2 2 2
  line L180 (2.207, 2.32) -> (2.207, 1.8257)
  line L181 (2.207, 1.8257) -> (2.0806, 1.8257)
  line L182 (-1.0945, 7.3327) -> (-1.7112, 7.3327)
  line L183 (-1.7112, 7.3327) -> (-1.7112, 7.4745)
  spline S172 degree 2 poles (-1.7112, 7.4745) (-1.6448, 7.5369) (-1.5264, 7.6528) (-1.4697, 7.7152) knots 0 0 0 1 2 2 2
  spline S173 degree 2 poles (-1.4697, 7.7152) (-1.3554, 7.8408) (-1.272, 7.9915) (-1.272, 8.0717) knots 0 0 0 1 2 2 2
  spline S174 degree 2 poles (-1.272, 8.0717) (-1.272, 8.1139) (-1.2979, 8.1771) (-1.3214, 8.1973) knots 0 0 0 1 2 2 2
  spline S175 degree 2 poles (-1.3214, 8.1973) (-1.3449, 8.2176) (-1.4065, 8.2378) (-1.4438, 8.2378) knots 0 0 0 1 2 2 2
  spline S176 degree 2 poles (-1.4438, 8.2378) (-1.4794, 8.2378) (-1.5524, 8.22) (-1.5856, 8.2062) knots 0 0 0 1 2 2 2
  spline S177 degree 2 poles (-1.5856, 8.2062) (-1.614, 8.1949) (-1.6666, 8.1625) (-1.6828, 8.1511) knots 0 0 0 1 2 2 2
  line L184 (-1.6828, 8.1511) -> (-1.6901, 8.1511)
  line L185 (-1.6901, 8.1511) -> (-1.6901, 8.2938)
  spline S178 degree 2 poles (-1.6901, 8.2938) (-1.6488, 8.314) (-1.5005, 8.3537) (-1.4341, 8.3537) knots 0 0 0 1 2 2 2
  spline S179 degree 2 poles (-1.4341, 8.3537) (-1.2939, 8.3537) (-1.1358, 8.2054) (-1.1358, 8.079) knots 0 0 0 1 2 2 2
  spline S180 degree 2 poles (-1.1358, 8.079) (-1.1358, 8.0199) (-1.1634, 7.921) (-1.1877, 7.8789) knots 0 0 0 1 2 2 2
  spline S181 degree 2 poles (-1.1877, 7.8789) (-1.212, 7.8351) (-1.2825, 7.7492) (-1.3214, 7.7079) knots 0 0 0 1 2 2 2
  spline S182 degree 2 poles (-1.3214, 7.7079) (-1.3846, 7.639) (-1.5394, 7.4915) (-1.5856, 7.4485) knots 0 0 0 1 2 2 2
  line L186 (-1.5856, 7.4485) -> (-1.0945, 7.4485)
  line L187 (-1.0945, 7.4485) -> (-1.0945, 7.3327)
  line L188 (-0.746, 7.3327) -> (-0.9065, 7.3327)
  line L189 (-0.9065, 7.3327) -> (-0.9065, 7.5239)
  line L190 (-0.9065, 7.5239) -> (-0.746, 7.5239)
  line L191 (-0.746, 7.5239) -> (-0.746, 7.3327)
  spline S183 degree 2 poles (-0.242, 7.31) (-0.3166, 7.31) (-0.4389, 7.3545) (-0.4819, 7.3959) knots 0 0 0 1 2 2 2
  spline S184 degree 2 poles (-0.4819, 7.3959) (-0.524, 7.4364) (-0.5678, 7.5466) (-0.5678, 7.609) knots 0 0 0 1 2 2 2
  spline S185 degree 2 poles (-0.5678, 7.609) (-0.5678, 7.69) (-0.4811, 7.8262) (-0.3984, 7.8667) knots 0 0 0 1 2 2 2
  line L192 (-0.3984, 7.8667) -> (-0.3984, 7.8708)
  spline S186 degree 2 poles (-0.3984, 7.8708) (-0.4721, 7.9137) (-0.5435, 8.0158) (-0.5435, 8.092) knots 0 0 0 1 2 2 2
  spline S187 degree 2 poles (-0.5435, 8.092) (-0.5435, 8.2046) (-0.3733, 8.3554) (-0.242, 8.3554) knots 0 0 0 1 2 2 2
  spline S188 degree 2 poles (-0.242, 8.3554) (-0.1059, 8.3554) (0.0587, 8.2127) (0.0587, 8.1009) knots 0 0 0 1 2 2 2
  spline S189 degree 2 poles (0.0587, 8.1009) (0.0587, 8.0336) (-0.02, 7.9024) (-0.0937, 7.8651) knots 0 0 0 1 2 2 2
  line L193 (-0.0937, 7.8651) -> (-0.0937, 7.861)
  spline S190 degree 2 poles (-0.0937, 7.861) (-0.0062, 7.8205) (0.0838, 7.7038) (0.0838, 7.6114) knots 0 0 0 1 2 2 2
  spline S191 degree 2 poles (0.0838, 7.6114) (0.0838, 7.4834) (-0.1026, 7.31) (-0.242, 7.31) knots 0 0 0 1 2 2 2
  spline S192 degree 2 poles (-0.054, 7.5985) (-0.054, 7.6601) (-0.1026, 7.733) (-0.1715, 7.7703) knots 0 0 0 1 2 2 2
  spline S193 degree 2 poles (-0.1715, 7.7703) (-0.1942, 7.7832) (-0.2704, 7.8132) (-0.3182, 7.8327) knots 0 0 0 1 2 2 2
  spline S194 degree 2 poles (-0.3182, 7.8327) (-0.3733, 7.7962) (-0.4324, 7.6876) (-0.4324, 7.6187) knots 0 0 0 1 2 2 2
  spline S195 degree 2 poles (-0.4324, 7.6187) (-0.4324, 7.528) (-0.323, 7.4096) (-0.2404, 7.4096) knots 0 0 0 1 2 2 2
  spline S196 degree 2 poles (-0.2404, 7.4096) (-0.1561, 7.4096) (-0.054, 7.5109) (-0.054, 7.5985) knots 0 0 0 1 2 2 2
  spline S197 degree 2 poles (-0.0726, 8.0993) (-0.0726, 8.1665) (-0.1626, 8.2565) (-0.2428, 8.2565) knots 0 0 0 1 2 2 2
  spline S198 degree 2 poles (-0.2428, 8.2565) (-0.3157, 8.2565) (-0.4089, 8.1763) (-0.4089, 8.1074) knots 0 0 0 1 2 2 2
  spline S199 degree 2 poles (-0.4089, 8.1074) (-0.4089, 8.0579) (-0.3611, 7.9891) (-0.3133, 7.9615) knots 0 0 0 1 2 2 2
  spline S200 degree 2 poles (-0.3133, 7.9615) (-0.293, 7.9502) (-0.2072, 7.9105) (-0.1723, 7.8991) knots 0 0 0 1 2 2 2
  spline S201 degree 2 poles (-0.1723, 7.8991) (-0.114, 7.9437) (-0.0726, 8.0385) (-0.0726, 8.0993) knots 0 0 0 1 2 2 2
  line L194 (1.0757, 7.3327) -> (1.0757, 7.767)
  spline S202 degree 2 poles (1.0757, 7.767) (1.0757, 7.8189) (1.0676, 7.9072) (1.0546, 7.9315) knots 0 0 0 1 2 2 2
  spline S203 degree 2 poles (1.0546, 7.9315) (1.0416, 7.9583) (0.9922, 7.9842) (0.9493, 7.9842) knots 0 0 0 1 2 2 2
  spline S204 degree 2 poles (0.9493, 7.9842) (0.9104, 7.9842) (0.8212, 7.9364) (0.7742, 7.891) knots 0 0 0 1 2 2 2
  spline S205 degree 2 poles (0.7742, 7.891) (0.775, 7.8797) (0.7766, 7.8481) (0.7766, 7.827) knots 0 0 0 1 2 2 2
  line L195 (0.7766, 7.827) -> (0.7766, 7.3327)
  line L196 (0.7766, 7.3327) -> (0.6502, 7.3327)
  line L197 (0.6502, 7.3327) -> (0.6502, 7.767)
  spline S206 degree 2 poles (0.6502, 7.767) (0.6502, 7.8189) (0.6421, 7.9072) (0.6292, 7.9315) knots 0 0 0 1 2 2 2
  spline S207 degree 2 poles (0.6292, 7.9315) (0.6162, 7.9583) (0.5668, 7.9842) (0.5238, 7.9842) knots 0 0 0 1 2 2 2
  spline S208 degree 2 poles (0.5238, 7.9842) (0.4833, 7.9842) (0.3933, 7.9331) (0.3512, 7.8934) knots 0 0 0 1 2 2 2
  line L198 (0.3512, 7.8934) -> (0.3512, 7.3327)
  line L199 (0.3512, 7.3327) -> (0.2248, 7.3327)
  line L200 (0.2248, 7.3327) -> (0.2248, 8.0831)
  line L201 (0.2248, 8.0831) -> (0.3512, 8.0831)
  line L202 (0.3512, 8.0831) -> (0.3512, 8.0004)
  spline S209 degree 2 poles (0.3512, 8.0004) (0.4006, 8.0498) (0.4979, 8.1041) (0.5562, 8.1041) knots 0 0 0 1 2 2 2
  spline S210 degree 2 poles (0.5562, 8.1041) (0.6227, 8.1041) (0.7256, 8.0434) (0.7523, 7.9745) knots 0 0 0 1 2 2 2
  spline S211 degree 2 poles (0.7523, 7.9745) (0.8099, 8.0385) (0.9185, 8.1041) (0.9817, 8.1041) knots 0 0 0 1 2 2 2
  spline S212 degree 2 poles (0.9817, 8.1041) (1.0303, 8.1041) (1.1097, 8.0742) (1.1389, 8.0401) knots 0 0 0 1 2 2 2
  spline S213 degree 2 poles (1.1389, 8.0401) (1.1689, 8.0061) (1.2021, 7.904) (1.2021, 7.827) knots 0 0 0 1 2 2 2
  line L203 (1.2021, 7.827) -> (1.2021, 7.3327)
  line L204 (1.2021, 7.3327) -> (1.0757, 7.3327)
  line L205 (2.2305, 7.3327) -> (2.2305, 7.767)
  spline S214 degree 2 poles (2.2305, 7.767) (2.2305, 7.8189) (2.2223, 7.9072) (2.2094, 7.9315) knots 0 0 0 1 2 2 2
  spline S215 degree 2 poles (2.2094, 7.9315) (2.1964, 7.9583) (2.147, 7.9842) (2.104, 7.9842) knots 0 0 0 1 2 2 2
  spline S216 degree 2 poles (2.104, 7.9842) (2.0651, 7.9842) (1.976, 7.9364) (1.929, 7.891) knots 0 0 0 1 2 2 2
  spline S217 degree 2 poles (1.929, 7.891) (1.9298, 7.8797) (1.9314, 7.8481) (1.9314, 7.827) knots 0 0 0 1 2 2 2
  line L206 (1.9314, 7.827) -> (1.9314, 7.3327)
  line L207 (1.9314, 7.3327) -> (1.805, 7.3327)
  line L208 (1.805, 7.3327) -> (1.805, 7.767)
  spline S218 degree 2 poles (1.805, 7.767) (1.805, 7.8189) (1.7969, 7.9072) (1.7839, 7.9315) knots 0 0 0 1 2 2 2
  spline S219 degree 2 poles (1.7839, 7.9315) (1.771, 7.9583) (1.7215, 7.9842) (1.6786, 7.9842) knots 0 0 0 1 2 2 2
  spline S220 degree 2 poles (1.6786, 7.9842) (1.6381, 7.9842) (1.5481, 7.9331) (1.506, 7.8934) knots 0 0 0 1 2 2 2
  line L209 (1.506, 7.8934) -> (1.506, 7.3327)
  line L210 (1.506, 7.3327) -> (1.3796, 7.3327)
  line L211 (1.3796, 7.3327) -> (1.3796, 8.0831)
  line L212 (1.3796, 8.0831) -> (1.506, 8.0831)
  line L213 (1.506, 8.0831) -> (1.506, 8.0004)
  spline S221 degree 2 poles (1.506, 8.0004) (1.5554, 8.0498) (1.6527, 8.1041) (1.711, 8.1041) knots 0 0 0 1 2 2 2
  spline S222 degree 2 poles (1.711, 8.1041) (1.7775, 8.1041) (1.8804, 8.0434) (1.9071, 7.9745) knots 0 0 0 1 2 2 2
  spline S223 degree 2 poles (1.9071, 7.9745) (1.9646, 8.0385) (2.0732, 8.1041) (2.1364, 8.1041) knots 0 0 0 1 2 2 2
  spline S224 degree 2 poles (2.1364, 8.1041) (2.1851, 8.1041) (2.2645, 8.0742) (2.2937, 8.0401) knots 0 0 0 1 2 2 2
  spline S225 degree 2 poles (2.2937, 8.0401) (2.3236, 8.0061) (2.3569, 7.904) (2.3569, 7.827) knots 0 0 0 1 2 2 2
  line L214 (2.3569, 7.827) -> (2.3569, 7.3327)
  line L215 (2.3569, 7.3327) -> (2.2305, 7.3327)
  point P0 (0, 0)
  constraints: 11 other
extrude "Extrusion2" cut sketch "Sketch2" against normal blind 2
equation "\"d2\" = d1"
equation "\"d5\" = d1"
equation "\"d6\" = d2"
body "Solid1"
